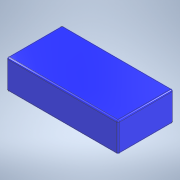
# Autodesk Inventor part: Battery[72x36x19]
Saved by Autodesk Inventor 2020 (Build 240168000, 168)
## iProperties
Created: 2019-12-14
Part Number: Battery[72x36x19]
Material: Generic
Document SubType Name: Modeling
Designer: ermoz
Density: 1 g/cm^3
Appearance: Default
Mass: 49.1403 g
Surface Area: 90.6883 cm^2
Volume: 49.1403 cm^3
Author: ermoz
Autodesk Inventor part; units mm, degrees
ref_plane "YZ Plane" through (0, 0, 0) normal (1, 0, 0) x (0, 1, 0)
ref_plane "XZ Plane" through (0, 0, 0) normal (0, 1, 0) x (-1, 0, 0)
ref_plane "XY Plane" through (0, 0, 0) normal (0, 0, 1) x (1, 0, 0)
sketch "Sketch1" plane through (0, 0, 0) normal (0, 1, 0) x (-1, 0, 0)
  line L0 (0, 0) -> (72, 0)
  line L1 (72, 0) -> (72, -36)
  line L2 (72, -36) -> (0, -36)
  line L3 (0, -36) -> (0, 0)
  dimension "d0" = 72
  dimension "d1" = 36
  constraints: 8 end point, 2 parallel, 1 horizontal, 1 perpendicular
  measures "d0" distance of L1.end L2.end
  measures "d1" distance of L0.end L1.end
extrude "Extrusion1" add sketch "Sketch1" along normal blind 19
fillet "Fillet1" radius 1 12 edges at (0, 19, -18) (0, 0, -18) (0, 9.5, -36) (-36, 0, -36) (-36, 19, -36) (-72, 9.5, -36) (-72, 19, -18) (-72, 0, -18) (-72, 9.5, 0) (-36, 19, 0) (-36, 0, 0) (0, 9.5, 0)
body "Solid1"
